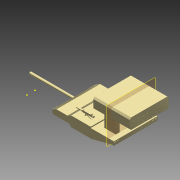
# Autodesk Inventor part: New Cannon M117 Guardian
Saved by Autodesk Inventor 2015 (Build 190159000, 159)
## iProperties
Created: 2015-04-16
Part Number: New Cannon M117 Guardian
Material: Generic
Document SubType Name: Modeling
Designer: AJ
Density: 1 g/cm^3
Appearance: Gold - Metal
Mass: 148.027 g
Surface Area: 618.94 cm^2
Volume: 148.027 cm^3
Author: AJ
Autodesk Inventor part; units mm, degrees
ref_plane "YZ Plane" through (0, 0, 0) normal (1, 0, 0) x (0, 1, 0)
ref_plane "XZ Plane" through (0, 0, 0) normal (0, 1, 0) x (-1, 0, 0)
sketch "Sketch1" plane through (0, 0, 0) normal (0, 0, 1) x (1, 0, 0)
  line L0 (-65.2349, 84.567) -> (296.1859, 84.567) construction
  line L1 (296.1859, 84.567) -> (296.1859, -118.633) construction
  line L2 (296.1859, -118.633) -> (-65.2349, -118.633) construction
  line L3 (-65.2349, -118.633) -> (-65.2349, 84.567) construction
  line L4 (147.7613, -1.0221) -> (112.6147, -10.0058)
  line L5 (112.6147, -10.0058) -> (77.1528, -10.0058)
  line L6 (77.1528, -10.0058) -> (70.6909, -2.4406)
  line L7 (70.6909, -2.4406) -> (77.1528, 5.755)
  line L8 (77.1528, 5.755) -> (147.7613, 5.755)
  line L9 (147.7613, 5.755) -> (151.5439, 5.755)
  line L10 (151.5439, 5.755) -> (151.5439, -1.0221)
  line L11 (151.5439, -1.0221) -> (149.6526, -0.5387)
  line L12 (70.6909, -2.4406) -> (87.5473, -2.4406)
  line L13 (87.5473, -2.4406) -> (87.5473, -10.0058)
  line L14 (77.1528, -10.0058) -> (87.5473, -2.4406)
  line L15 (111.1962, 5.755) -> (111.1962, 7.6463)
  line L16 (111.1962, 7.6463) -> (77.1528, 7.6463)
  line L17 (149.6526, -0.5387) -> (147.7613, -1.0221)
  line L18 (77.1528, 7.6463) -> (77.1528, 5.755)
  line L19 (77.1528, 7.6463) -> (70.6909, 4.2047)
  line L20 (70.6909, 4.2047) -> (51.5765, 4.2047)
  line L21 (51.5765, 4.2047) -> (44.322, 0.341)
  line L22 (44.322, 0.341) -> (44.322, -4.3674)
  line L23 (44.322, -4.3674) -> (45.7533, -6.2232)
  line L24 (45.7533, -6.2232) -> (73.9219, -6.2232)
  point P0 (0, 0)
  constraints: 42 end point, 6 perpendicular, 5 point on line, 2 horizontal, 2 parallel, 2 vertical, 1 collinear, 1 midpoint, 2 other
extrude "Extrusion1" add sketch "Sketch1" along normal blind 76.2
sketch "Sketch2" plane through (44.322, -4.3674, 0) normal (-1, 0, 0) x (0, 0, 1)
  line L0 (0, 4.7084) -> (76.2, 4.7084) projected
  line L1 (0, 0) -> (76.2, 0) projected
  line L2 (0, 4.7084) -> (0, 0) projected
  line L3 (0, 2.3542) -> (38.1, 2.3542)
  line L4 (76.2, 4.7084) -> (76.2, 0) projected
  circle A0 centre (38.1, 2.3542) radius 2.3542
  point P0 (0, 4.3674)
  dimension "d5" = 38.1
  constraints: 2 end point, 1 centre point, 1 coincident, 1 midpoint, 1 perpendicular
  measures "d5" distance of L3.start L3.end
extrude "Extrusion2" add sketch "Sketch2" along normal blind 76.2 contours A0
sketch "Sketch4" plane through (77.1528, -10.0058, 0) normal (0, -1, 0) x (1, 0, 0)
  line L0 (0, 0) -> (35.4619, 0) projected
  line L1 (35.4619, 0) -> (35.4619, 76.2) projected
  line L2 (0, 76.2) -> (35.4619, 76.2) projected
  line L3 (0, 0) -> (0, 76.2) projected
  line L4 (34.0434, 76.2) -> (0, 76.2) projected
  line L5 (0, 0) -> (35.4619, 0) projected
  line L6 (17.7309, 0) -> (17.7309, 76.2)
  line L7 (0, 76.2) -> (35.4619, 76.2) projected
  line L8 (35.4619, 0) -> (35.4619, 76.2) projected
  line L9 (35.4619, 38.1) -> (0, 38.1)
  point P0 (-77.1528, 0)
  point P1 (17.7309, 38.1)
  point P2 (17.7309, 38.1)
  point P3 (17.7309, 38.1)
  point P4 (17.7309, 38.1)
  point P5 (17.7309, 38.1)
  point P6 (17.7309, 38.1)
  constraints: 5 coincident, 5 midpoint, 4 end point
sketch "Sketch5" plane through (70.6909, 4.2047, 76.2) normal (-0.4700833, 0.8826221, 0) x (0.8826221, 0.4700833, 0)
  line L0 (37.3687, 76.2) -> (7.3213, 76.2) projected
  line L1 (7.3213, 76.2) -> (7.3213, 0) projected
  line L2 (37.3687, 0) -> (7.3213, 0) projected
  line L3 (37.3687, 76.2) -> (37.3687, 0) projected
  point P0 (-64.3699, 76.2)
hole "Hole2" at (94.8838, -10.0058, 38.1) direction (0, 1, 0) diameter 9.144 depth 9.271
ref_plane "Work Plane2" through (94.8838, -10.0058, 61.9125) normal (0, 0, 1) x (1, 0, 0)
ref_plane "Work Plane1" through (94.8838, -10.0058, 76.2) normal (0, 0, 1) x (1, 0, 0)
sketch "Sketch7" plane through (94.8838, -10.0058, 61.9125) normal (0, 0, 1) x (1, 0, 0)
  line L0 (16.3125, 17.6521) -> (-17.7309, 17.6521) projected
  line L1 (-6.0206, 17.6521) -> (-4.2827, 20.7702)
  line L2 (-2.8607, 20.7702) -> (-4.5987, 17.6521)
  line L3 (-2.8607, 20.7702) -> (-4.2827, 20.7702)
  line L4 (7.2447, 17.6521) -> (-2.8607, 20.7702)
  line L5 (-3.1978, 20.1656) -> (4.2174, 17.6521)
  line L6 (-4.2827, 20.7702) -> (-6.8227, 20.7702)
  arc A0 (-12.1362, 21.8532) -> (-6.8227, 20.7702) centre (-7.8983, 29.069) ccw
  line L7 (-12.1362, 21.8532) -> (-20.7565, 21.8532)
  line L8 (-20.7565, 21.8532) -> (-20.7565, 23.0624)
  line L9 (-20.7565, 23.0624) -> (-11.7414, 23.0624)
  arc A1 (-11.7414, 23.0624) -> (-8.8103, 24.103) centre (-11.7414, 27.7104) ccw
  line L10 (-8.8103, 24.103) -> (5.0635, 24.103)
  arc A2 (5.0635, 24.103) -> (9.0378, 23.4542) centre (7.3609, 25.6785) ccw
  line L11 (9.0378, 23.4542) -> (9.0378, 21.1026)
  arc A3 (9.0378, 21.1026) -> (5.0635, 21.1664) centre (6.935, 13.9229) ccw
  line L12 (5.0635, 21.1664) -> (-2.8607, 20.7702)
  line L13 (4.9167, 24.103) -> (4.9167, 24.6631)
  line L14 (4.9167, 24.103) -> (6.0369, 24.103) construction
  line L15 (-8.8103, 24.6631) -> (-8.8103, 24.103)
  line L16 (-8.3522, 24.6631) -> (-8.3522, 24.103)
  line L17 (4.3443, 24.6631) -> (4.3443, 24.103)
  line L18 (4.9167, 24.6631) -> (4.3443, 24.6631)
  line L19 (-8.3522, 24.6631) -> (-8.8103, 24.6631)
  point P0 (-94.8838, 10.0058)
  dimension "d27" = 2.54
  dimension "d28" = 90
  constraints: 38 end point, 9 point on line, 8 point on circle, 7 horizontal, 5 perpendicular, 4 centre point, 2 vertical, 1 tangent
  measures "d27" distance of L3.end L6.end
  measures "d28" angle of L14 L13
extrude "Extrusion3" add sketch "Sketch7" along normal blind 2.54 contours L0 L5 L2 L4 | L2 L0 L1 L3 | L3 L6 A0 L7 L8 L9 A1 L10 A2 L11 A3 L12 | L10 L17 L18 L13 | L15 L19 L16 L10
ref_plane "Work Plane3" through (94.8838, -10.0058, 39.6875) normal (0, 0, 1) x (1, 0, 0)
mirror "Mirror1" about plane through (94.8838, -10.0058, 39.6875) normal (0, 0, 1) of "Extrusion3"
sketch "Sketch9" plane through (94.8838, -10.0058, 61.9125) normal (0, 0, 1) x (1, 0, 0)
  point P0 (-94.8838, 10.0058)
sketch "Sketch10" plane through (0, 0, 76.2) normal (0, 0, 1) x (1, 0, 0)
  point P0 (0, 0)
sketch "Sketch11" plane through (111.1962, 5.755, 0) normal (0, 1, 0) x (1, 0, 0)
  line L0 (11.9426, -64.0725) -> (31.6954, -64.0725)
  line L1 (40.3477, -76.2) -> (0, -76.2) projected
  line L2 (11.9426, -12.1158) -> (31.6954, -12.1158)
  line L3 (40.3477, 0) -> (0, 0) projected
  line L4 (11.9426, -64.0725) -> (11.9426, -12.1158)
  line L5 (31.6954, -12.1158) -> (31.6954, -64.0725)
  line L6 (11.9426, -57.2907) -> (31.6954, -57.2907)
  line L7 (31.6954, -18.9064) -> (11.9426, -18.9064)
  point P0 (-111.1962, 0)
  dimension "d34" = 12.1275
  dimension "d35" = 12.1158
  dimension "d36" = 6.7906
  dimension "d37" = 6.7818
  constraints: 12 end point, 4 point on line, 2 horizontal, 2 perpendicular, 1 parallel, 1 vertical
  measures "d34" distance between parallel lines of L1 L0
  measures "d35" distance between parallel lines of L3 L2
  measures "d36" distance between parallel lines of L2 L7
  measures "d37" distance between parallel lines of L0 L6
extrude "Extrusion4" add sketch "Sketch11" along normal blind 25.4 contours L4 L6 L5 L0 | L4 L2 L5 L7
ref_plane "Work Plane4" through (142.8916, 18.455, 64.0725) normal (1, 0, 0) x (0, 0, -1)
sketch "Sketch12" plane through (142.8916, 18.455, 64.0725) normal (1, 0, 0) x (0, 0, -1)
  line L0 (-7.7087, 31.4594) -> (55.7913, 31.4594)
  line L1 (-7.7087, 31.4594) -> (-7.7087, 12.6385)
  line L2 (-7.7087, 12.6385) -> (57.4494, 12.6385)
  line L3 (-7.7087, 22.049) -> (57.4494, 22.049)
  line L4 (0.836, 31.4594) -> (0.836, 12.7)
  line L5 (0, 12.7) -> (6.7818, 12.7) projected
  line L6 (0.836, 31.4594) -> (9.3704, 31.4594)
  line L7 (9.3704, 31.4594) -> (9.3704, 12.6385)
  line L8 (9.3704, 31.4594) -> (17.9048, 31.4594)
  line L9 (17.9048, 31.4594) -> (17.9048, 12.6385)
  line L10 (17.9048, 31.4594) -> (26.4392, 31.4594)
  line L11 (26.4392, 31.4594) -> (26.4392, 12.6385)
  line L12 (26.4392, 31.4594) -> (34.9736, 31.4594)
  line L13 (34.9736, 31.4594) -> (34.9736, 12.6385)
  line L14 (34.9736, 31.4594) -> (43.508, 31.4594)
  line L15 (43.508, 31.4594) -> (52.0424, 31.4594)
  line L16 (52.0424, 31.4594) -> (52.0424, 12.6385)
  line L17 (52.0424, 31.4594) -> (60.5768, 31.4594)
  line L18 (60.5768, 31.4594) -> (60.5768, 12.6385)
  line L19 (60.5768, 12.6385) -> (57.4494, 12.6385)
  line L20 (57.4494, 22.049) -> (60.5768, 22.049)
  line L21 (45.1661, -12.7) -> (45.1661, 12.7) projected
  line L22 (43.508, 31.4594) -> (43.508, 12.6385)
  line L23 (60.5768, 31.4594) -> (56.3096, 31.4594)
  line L24 (56.3096, 31.4594) -> (56.3096, 26.7604)
  circle A0 centre (56.3096, 26.7604) radius 4.0218
  circle A1 centre (47.7752, 26.7604) radius 4.0218
  circle A2 centre (39.2408, 26.7604) radius 4.0218
  circle A3 centre (30.7064, 26.7604) radius 4.0218
  circle A4 centre (22.172, 26.7604) radius 4.0218
  circle A5 centre (13.6376, 26.7604) radius 4.0218
  circle A6 centre (5.1032, 26.7604) radius 4.0218
  circle A7 centre (-3.4114, 26.7604) radius 4.0261
  line L25 (56.3096, 17.35) -> (60.5768, 17.35)
  circle A8 centre (47.7752, 17.35) radius 4.005
  circle A9 centre (39.2408, 17.35) radius 4.0574
  circle A10 centre (30.7064, 17.35) radius 4.0574
  circle A11 centre (22.172, 17.35) radius 4.0452
  circle A12 centre (13.6376, 17.35) radius 4.0795
  circle A13 centre (5.1032, 17.35) radius 4.0795
  point P0 (64.0725, -18.455)
  dimension "d42" = 63.5
  dimension "d43" = 8.5448
  dimension "d44" = 8.5344
  dimension "d45" = 8.5344
  dimension "d46" = 8.5344
  dimension "d47" = 8.5344
  dimension "d48" = 8.5344
  dimension "d49" = 8.5344
  dimension "d50" = 8.5344
  dimension "d51" = 4.2672
  dimension "d52" = 4.699
  constraints: 46 end point, 14 centre point, 10 perpendicular, 8 point on line, 3 midpoint, 3 vertical, 1 coincident, 1 horizontal, 10 other
  measures "d42" distance of L1.start point (55.791, 31.459)
  measures "d43" distance between parallel lines of L1 L4
  measures "d44" distance of L4.start L6.end
  measures "d45" distance of L6.end L8.end
  measures "d46" distance of L8.end L10.end
  measures "d47" distance of L10.end L12.end
  measures "d48" distance of L12.end L14.end
  measures "d49" distance of L14.end L15.end
  measures "d50" distance of L15.end L17.end
  measures "d51" distance of L17.end L23.end
  measures "d52" distance of L23.end L24.end
extrude "Extrusion5" add sketch "Sketch12" along normal mid plane 63.5
chamfer "Chamfer1" distance 2.54 angle 45 4 edges at (142.8916, 49.9144, 71.7813) (142.8916, 49.9144, 3.4957) (142.8916, 31.0935, 3.4957) (142.8916, 31.0935, 71.7813)
sketch "Sketch13" plane through (174.6416, 18.455, 64.0725) normal (1, 0, 0) x (0, 0, -1)
  line L0 (-5.1687, 31.4594) -> (-7.7311, 28.8715)
  line L1 (-7.7311, 28.8715) -> (-7.7311, 15.2009)
  line L2 (58.0368, 31.4594) -> (-5.1687, 31.4594) projected
  line L3 (-7.7311, 15.2009) -> (-5.1687, 12.6385)
  line L4 (-5.1687, 12.6385) -> (-7.7087, 15.1785) projected
  line L5 (-5.1687, 12.6385) -> (58.0368, 12.6385)
  line L6 (58.0368, 12.6385) -> (60.5768, 15.1785)
  line L7 (60.5768, 15.1785) -> (58.0368, 12.6385) projected
  line L8 (60.5768, 15.1785) -> (60.5768, 28.8715)
  line L9 (60.5768, 28.8715) -> (58.0368, 31.4594)
  line L10 (58.0368, 31.4594) -> (60.5768, 28.9194) projected
  point P0 (64.0725, -18.455)
  constraints: 14 end point, 3 perpendicular, 2 collinear, 1 point on line
extrude "Extrusion6" add sketch "Sketch13" along normal blind 0.0254
sketch "Sketch14" plane through (151.5439, -1.0221, 0) normal (1, 0, 0) x (0, 0, -1)
  line L0 (0, 0) -> (0, 6.7772) projected
  line L1 (0, 6.7772) -> (-76.2, 6.7772) projected
  line L2 (-76.2, 0) -> (-76.2, 6.7772) projected
  line L3 (0, 0) -> (-76.2, 0) projected
  line L4 (-76.2, 6.7772) -> (-66.04, 6.7772)
  line L5 (0, 6.7772) -> (-76.2, 6.7772) projected
  line L6 (0, 6.7772) -> (-10.16, 6.7772)
  line L7 (-10.16, 6.7772) -> (-5.08, 6.7772)
  line L8 (-76.2, 6.7772) -> (-71.12, 6.7772)
  line L9 (-71.12, 6.7772) -> (-71.12, 0)
  line L10 (-76.2, 0.4834) -> (-76.2, 6.7772)
  line L11 (0, 0.4834) -> (-76.2, 0.4834) projected
  line L12 (-66.04, 6.7772) -> (-66.04, 0.4834)
  line L13 (-10.16, 6.7772) -> (-10.16, 0)
  line L14 (0, 0) -> (-76.2, 0) projected
  line L15 (-5.08, 0) -> (-5.08, 6.7772)
  line L16 (0, 0) -> (-5.08, 0)
  line L17 (-66.04, 0.4834) -> (-66.04, 0)
  line L18 (-76.2, 3.3886) -> (0, 3.3886)
  circle A0 centre (-73.66, 3.3886) radius 1.9406
  circle A1 centre (-68.5548, 3.3886) radius 2.0416
  circle A2 centre (-7.62, 3.3886) radius 1.9406
  circle A3 centre (-2.54, 3.3886) radius 1.9406
  point P0 (0, 1.0221)
  dimension "d61" = 10.16
  dimension "d62" = 10.16
  dimension "d63" = 5.08
  dimension "d64" = 5.08
  constraints: 24 end point, 13 point on line, 6 perpendicular, 4 centre point, 2 midpoint, 1 collinear
  measures "d61" distance of L1.end L4.end
  measures "d62" distance of L0.end L6.end
  measures "d63" distance of L6.end L7.end
  measures "d64" distance of L1.end L8.end
extrude "Extrusion7" add sketch "Sketch14" along normal blind 0.762 contours A3 L18 | L18 A3 | A2 L18 | L18 A2 | A1 L18 | L18 A1 | A0 L18 | L18 A0
sketch "Sketch15" plane through (44.322, -4.3674, 0) normal (-1, 0, 0) x (0, 0, 1)
  arc A0 (38.1, 4.7084) -> (38.1, 0) centre (38.1, 2.3542) ccw projected
  line L0 (0, 4.7084) -> (38.1, 4.7084) projected
  line L1 (0, 4.7084) -> (0, 0) projected
  line L2 (0, 0) -> (38.1, 0) projected
  arc A1 (38.1, 0) -> (38.1, 4.7084) centre (38.1, 2.3542) ccw projected
  line L3 (38.1, 0) -> (76.2, 0) projected
  line L4 (76.2, 4.7084) -> (76.2, 0) projected
  line L5 (38.1, 4.7084) -> (76.2, 4.7084) projected
  circle A2 centre (38.1, 2.3542) radius 2.3542 projected
  line L6 (0, 4.7084) -> (10.16, 4.7084)
  line L7 (10.16, 4.7084) -> (10.16, 0)
  line L8 (0, 0) -> (38.1, 0) projected
  line L9 (5.08, 0) -> (5.08, 4.7084)
  line L10 (76.2, 4.7084) -> (66.04, 4.7084)
  line L11 (66.04, 4.7084) -> (66.04, 0)
  line L12 (38.1, 0) -> (76.2, 0) projected
  line L13 (71.12, 0) -> (71.12, 4.7084)
  line L14 (0, -5.6384) -> (0, 3.8287) projected
  line L15 (0, 2.3542) -> (76.2, 2.3542)
  circle A3 centre (2.4635, 2.3542) radius 2.0992
  circle A4 centre (7.8157, 2.3542) radius 2.0955
  circle A5 centre (68.558, 2.3542) radius 2.0955
  circle A6 centre (73.8712, 2.3542) radius 2.0955
  point P0 (0, 4.3674)
  dimension "d67" = 10.16
  dimension "d68" = 10.16
  dimension "d69" = 4.191
  dimension "d70" = 4.191
  dimension "d71" = 4.191
  constraints: 14 end point, 11 point on line, 4 centre point, 3 midpoint, 2 perpendicular
  measures "d67" distance of L0.start L6.end
  measures "d68" distance of L4.start L10.end
  measures "d69" diameter of A4
  measures "d70" diameter of A5
  measures "d71" diameter of A6
extrude "Extrusion8" add sketch "Sketch15" along normal blind 0.762 contours A4 L15 | L15 A4 | A5 L15 | L15 A5 | A3 L15 | L15 A3 | A6 L15 | L15 A6
sketch "Sketch16" plane through (-31.878, -2.0132, 38.1) normal (-1, 0, 0) x (0, 0, 1)
  circle A0 centre (0, 0) radius 2.3542 projected
  point P0 (-38.1, 2.0132)
  constraints: 1 coincident
hole "Hole3" at (-31.878, -2.0132, 38.1) direction (1, 0, 0) diameter 3.81 depth 96.52
body "Solid1"
